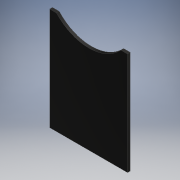
# Autodesk Inventor part: Electronics Plate
Saved by Autodesk Inventor 2017 (Build 210142000, 142)
## iProperties
Created: 2018-10-14
Part Number: Electronics Plate
Material: Generic
Document SubType Name: Modeling
Designer: Cameron
Density: 1 g/cm^3
Appearance: Glossy - Black
Author: Cameron
Autodesk Inventor part; units mm, degrees
ref_plane "YZ Plane" through (0, 0, 0) normal (1, 0, 0) x (0, 1, 0)
ref_plane "XZ Plane" through (0, 0, 0) normal (0, 1, 0) x (-1, 0, 0)
ref_plane "XY Plane" through (0, 0, 0) normal (0, 0, 1) x (1, 0, 0)
sketch "Sketch1" plane through (0, 0, 0) normal (0, 1, 0) x (-1, 0, 0)
  line L0 (85, 0) -> (85, -112)
  line L1 (85, -112) -> (0, -112)
  line L2 (0, -112) -> (0, 0)
  arc A0 (7.3966, 0) -> (77.6034, 0) centre (42.5, 32) ccw
  line L3 (0, 0) -> (7.3966, 0)
  line L4 (77.6034, 0) -> (85, 0)
  dimension "d0" = 112
  dimension "d1" = 85
  constraints: 10 end point, 3 parallel, 2 horizontal, 2 perpendicular, 2 point on circle, 1 centre point
  measures "d0" distance of L0.start L0.end
  measures "d1" distance between parallel lines of L2 L0
extrude "Extrusion1" add sketch "Sketch1" along normal blind 3
body "Solid1"
